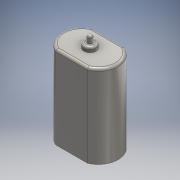
# Autodesk Inventor part: Motor
Saved by Autodesk Inventor 2016 (Build 200138000, 138)
## iProperties
Created: 2016-09-22
Part Number: Motor
Material: Acero inoxidable
Document SubType Name: Modeling
Designer: i95sa
Density: 8 g/cm^3
Appearance: Semipulido
Author: i95sa
Autodesk Inventor part; units mm, degrees
ref_plane "YZ Plane" through (0, 0, 0) normal (1, 0, 0) x (0, 1, 0)
ref_plane "XZ Plane" through (0, 0, 0) normal (0, 1, 0) x (-1, 0, 0)
ref_plane "XY Plane" through (0, 0, 0) normal (0, 0, 1) x (1, 0, 0)
sketch "Boceto1" plane through (0, 0, 0) normal (0, 0, 1) x (1, 0, 0)
  line L0 (0, 0) -> (6.5, 0)
  arc A0 (6.5, 0) -> (6.5, 15) centre (3.375, 7.5) ccw
  circle A1 centre (0, 7.5) radius 2.5
  line L1 (6.5, 15) -> (0, 15)
  circle A2 centre (0, 7.5) radius 5.0061
  line L2 (0, 0) -> (-6.5, 0)
  line L3 (0, 15) -> (-6.5, 15)
  arc A3 (-6.5, 15) -> (-6.5, 0) centre (-3.375, 7.5) ccw
  line L4 (0, 14.5653) -> (6.4118, 14.5653)
  arc A4 (6.4118, 0.4347) -> (6.4118, 14.5653) centre (3.375, 7.5) ccw
  line L5 (6.4118, 0.4347) -> (0, 0.4347)
  line L6 (0, 0.4347) -> (-6.4118, 0.4347)
  arc A5 (-6.4118, 14.5653) -> (-6.4118, 0.4347) centre (-3.375, 7.5) ccw
  line L7 (-6.4118, 14.5653) -> (0, 14.5653)
  dimension "d0" = 6.5
  dimension "d1" = 15
  dimension "d3" = 5
  dimension "d4" = 6.5
  constraints: 16 end point, 8 point on circle, 6 centre point, 3 horizontal, 1 coincident, 5 other
  measures "d0" distance of L0.start L0.end
  measures "d1" distance of L0.end L1.start
  measures "d3" diameter of A1
  measures "d4" distance of L0.start L2.end
extrude "Extrusión1" add sketch "Boceto1" along normal blind 33 contours L2 A3 L3 L1 A0 L0 | A1 | A2 | L4 A4 L5 L6 A5 L7
extrude "Extrusión2" add sketch "Boceto1" against normal blind 2 contours A1
extrude "Extrusión3" add sketch "Boceto1" against normal blind 1 contours A2
sketch "Boceto2" plane through (0, 0, 33) normal (0, 0, 1) x (1, 0, 0)
  line L0 (0, 0) -> (0, 15)
  line L1 (6.5, 15) -> (-6.5, 15) projected
  circle A0 centre (0, 7.5) radius 2.5
  circle A1 centre (0, 7.5) radius 1
  dimension "d12" = 5
  dimension "d13" = 2
  constraints: 2 centre point, 2 end point, 2 midpoint, 1 coincident
  measures "d12" diameter of A0
  measures "d13" diameter of A1
extrude "Extrusión4" add sketch "Boceto2" along normal blind 2 contours A0 L0 A1 | L0 A1 A0
extrude "Extrusión5" add sketch "Boceto2" along normal blind 5 contours A1 L0 | L0 A1
extrude "Extrusión6" add sketch "Boceto1" against normal blind 1 contours L2 A3 L3 L1 A0 L0
fillet "Empalme1" radius 1 8 edges at (-2.5, 7.5, -2) (-5.0061, 7.5, -1) (11.5, 7.5, 33) (0, 15, 33) (0, 0, 33) (-11.5, 7.5, 33) (-2.5, 7.5, 35) (-1, 7.5, 38)
